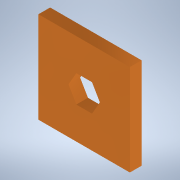
# Autodesk Inventor part: hex slot holder
Saved by Autodesk Inventor 2022 (Build 260153000, 153)
## iProperties
Created: 2021-05-28
Part Number: hex slot holder
Material: Gold
Document SubType Name: Modeling
Designer: benka
Density: 19.3 g/cm^3
Appearance: Metal 1600F Hot
Author: benka
Autodesk Inventor part; units mm, degrees
ref_plane "YZ Plane" through (0, 0, 0) normal (1, 0, 0) x (0, 1, 0)
ref_plane "XZ Plane" through (0, 0, 0) normal (0, 1, 0) x (-1, 0, 0)
ref_plane "XY Plane" through (0, 0, 0) normal (0, 0, 1) x (1, 0, 0)
sketch "Sketch1" plane through (0, 0, 0) normal (0, 0, 1) x (1, 0, 0)
  line L0 (-2.0207, 3.5005) -> (2.0207, 3.5005)
  line L1 (2.0207, 3.5005) -> (4.0415, 0.0005)
  line L2 (-4.0415, 0.0005) -> (-2.0207, 3.5005)
  line L3 (-2.0207, -3.4995) -> (-4.0415, 0.0005)
  line L4 (4.0415, 0.0005) -> (2.0207, -3.4995)
  line L5 (2.0207, -3.4995) -> (-2.0207, -3.4995)
  line L6 (-11.749, 11.7485) -> (11.751, 11.7485)
  line L7 (11.751, 11.7485) -> (11.751, -11.7515)
  line L8 (11.751, -11.7515) -> (-11.749, -11.7515)
  line L9 (-11.749, -11.7515) -> (-11.749, 11.7485)
  point P0 (0, 0)
  point P1 (0.001, -0.0015)
  dimension "d7" = 23.5
  dimension "d8" = 23.5
  constraints: 20 end point, 2 parallel, 1 horizontal, 1 perpendicular
  measures "d7" distance of L7.end L8.end
  measures "d8" distance of L6.end L7.end
extrude "Extrusion1" add sketch "Sketch1" along normal blind 3
body "Solid1"
